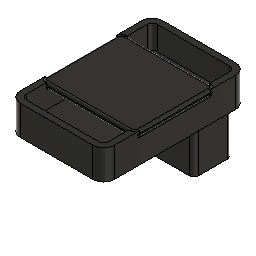
HX711mount (Autodesk Fusion 360 design; units mm, degrees)
Autodesk Fusion 360 part; units mm, degrees
sketch "Sketch1" plane through (0, 0, -6.0198) normal (0, 0, 1) x (-1, 0, 0)
  line L0 (-4.0409, -120.65) -> (2.9359, -120.65)
  line L1 (2.9359, -120.65) -> (3.9347, -119.6512)
  line L2 (3.9347, -119.6512) -> (3.9347, -58.1488)
  line L3 (3.9347, -58.1488) -> (2.9359, -57.15)
  line L4 (2.9359, -57.15) -> (3.9347, -56.1512)
  line L5 (3.9347, -56.1512) -> (3.9347, 6.35)
  line L6 (3.9347, 6.35) -> (-16.6393, 6.35)
  line L7 (-16.6393, 6.35) -> (-16.6393, -56.1512)
  line L8 (-16.6393, -56.1512) -> (-15.6405, -57.15)
  line L9 (-15.6405, -57.15) -> (-16.6393, -58.1488)
  line L10 (-16.6393, -58.1488) -> (-16.6393, -119.6512)
  line L11 (-16.6393, -119.6512) -> (-15.6405, -120.65)
  line L12 (-15.6405, -120.65) -> (-8.6637, -120.65)
  line L13 (-8.6637, -120.65) -> (-8.6637, -118.8466)
  arc A0 (-8.1557, -118.3386) -> (-8.6637, -118.8466) centre (-8.1557, -118.8466) ccw
  line L14 (-8.1557, -118.3386) -> (-4.5489, -118.3386)
  arc A1 (-4.0409, -118.8466) -> (-4.5489, -118.3386) centre (-4.5489, -118.8466) ccw
  line L15 (-4.0409, -118.8466) -> (-4.0409, -120.65)
  arc A2 (-8.1557, -105.6386) -> (-8.6637, -106.1466) centre (-8.1557, -106.1466) ccw
  line L16 (-8.1557, -105.6386) -> (-4.5489, -105.6386)
  arc A3 (-4.0409, -106.1466) -> (-4.5489, -105.6386) centre (-4.5489, -106.1466) ccw
  line L17 (-4.0409, -106.1466) -> (-4.0409, -109.7534)
  arc A4 (-4.5489, -110.2614) -> (-4.0409, -109.7534) centre (-4.5489, -109.7534) ccw
  line L18 (-4.5489, -110.2614) -> (-8.1557, -110.2614)
  arc A5 (-8.6637, -109.7534) -> (-8.1557, -110.2614) centre (-8.1557, -109.7534) ccw
  line L19 (-8.6637, -109.7534) -> (-8.6637, -106.1466)
  arc A6 (-8.1557, -92.9386) -> (-8.6637, -93.4466) centre (-8.1557, -93.4466) ccw
  line L20 (-8.1557, -92.9386) -> (-4.5489, -92.9386)
  arc A7 (-4.0409, -93.4466) -> (-4.5489, -92.9386) centre (-4.5489, -93.4466) ccw
  line L21 (-4.0409, -93.4466) -> (-4.0409, -97.0534)
  arc A8 (-4.5489, -97.5614) -> (-4.0409, -97.0534) centre (-4.5489, -97.0534) ccw
  line L22 (-4.5489, -97.5614) -> (-8.1557, -97.5614)
  arc A9 (-8.6637, -97.0534) -> (-8.1557, -97.5614) centre (-8.1557, -97.0534) ccw
  line L23 (-8.6637, -97.0534) -> (-8.6637, -93.4466)
  arc A10 (-8.1557, -80.2386) -> (-8.6637, -80.7466) centre (-8.1557, -80.7466) ccw
  line L24 (-8.1557, -80.2386) -> (-4.5489, -80.2386)
  arc A11 (-4.0409, -80.7466) -> (-4.5489, -80.2386) centre (-4.5489, -80.7466) ccw
  line L25 (-4.0409, -80.7466) -> (-4.0409, -84.3534)
  arc A12 (-4.5489, -84.8614) -> (-4.0409, -84.3534) centre (-4.5489, -84.3534) ccw
  line L26 (-4.5489, -84.8614) -> (-8.1557, -84.8614)
  arc A13 (-8.6637, -84.3534) -> (-8.1557, -84.8614) centre (-8.1557, -84.3534) ccw
  line L27 (-8.6637, -84.3534) -> (-8.6637, -80.7466)
  arc A14 (-8.1557, -67.5386) -> (-8.6637, -68.0466) centre (-8.1557, -68.0466) ccw
  line L28 (-8.1557, -67.5386) -> (-4.5489, -67.5386)
  arc A15 (-4.0409, -68.0466) -> (-4.5489, -67.5386) centre (-4.5489, -68.0466) ccw
  line L29 (-4.0409, -68.0466) -> (-4.0409, -71.6534)
  arc A16 (-4.5489, -72.1614) -> (-4.0409, -71.6534) centre (-4.5489, -71.6534) ccw
  line L30 (-4.5489, -72.1614) -> (-8.1557, -72.1614)
  arc A17 (-8.6637, -71.6534) -> (-8.1557, -72.1614) centre (-8.1557, -71.6534) ccw
  line L31 (-8.6637, -71.6534) -> (-8.6637, -68.0466)
  arc A18 (-8.1557, -54.8386) -> (-8.6637, -55.3466) centre (-8.1557, -55.3466) ccw
  line L32 (-8.1557, -54.8386) -> (-4.5489, -54.8386)
  arc A19 (-4.0409, -55.3466) -> (-4.5489, -54.8386) centre (-4.5489, -55.3466) ccw
  line L33 (-4.0409, -55.3466) -> (-4.0409, -58.9534)
  arc A20 (-4.5489, -59.4614) -> (-4.0409, -58.9534) centre (-4.5489, -58.9534) ccw
  line L34 (-4.5489, -59.4614) -> (-8.1557, -59.4614)
  arc A21 (-8.6637, -58.9534) -> (-8.1557, -59.4614) centre (-8.1557, -58.9534) ccw
  line L35 (-8.6637, -58.9534) -> (-8.6637, -55.3466)
  arc A22 (-8.1557, -42.1386) -> (-8.6637, -42.6466) centre (-8.1557, -42.6466) ccw
  line L36 (-8.1557, -42.1386) -> (-4.5489, -42.1386)
  arc A23 (-4.0409, -42.6466) -> (-4.5489, -42.1386) centre (-4.5489, -42.6466) ccw
  line L37 (-4.0409, -42.6466) -> (-4.0409, -46.2534)
  arc A24 (-4.5489, -46.7614) -> (-4.0409, -46.2534) centre (-4.5489, -46.2534) ccw
  line L38 (-4.5489, -46.7614) -> (-8.1557, -46.7614)
  arc A25 (-8.6637, -46.2534) -> (-8.1557, -46.7614) centre (-8.1557, -46.2534) ccw
  line L39 (-8.6637, -46.2534) -> (-8.6637, -42.6466)
  arc A26 (-8.1557, -29.4386) -> (-8.6637, -29.9466) centre (-8.1557, -29.9466) ccw
  line L40 (-8.1557, -29.4386) -> (-4.5489, -29.4386)
  arc A27 (-4.0409, -29.9466) -> (-4.5489, -29.4386) centre (-4.5489, -29.9466) ccw
  line L41 (-4.0409, -29.9466) -> (-4.0409, -33.5534)
  arc A28 (-4.5489, -34.0614) -> (-4.0409, -33.5534) centre (-4.5489, -33.5534) ccw
  line L42 (-4.5489, -34.0614) -> (-8.1557, -34.0614)
  arc A29 (-8.6637, -33.5534) -> (-8.1557, -34.0614) centre (-8.1557, -33.5534) ccw
  line L43 (-8.6637, -33.5534) -> (-8.6637, -29.9466)
  arc A30 (1.8011, -116.6114) -> (2.3091, -116.1034) centre (1.8011, -116.1034) ccw
  line L44 (1.8011, -116.6114) -> (-1.8057, -116.6114)
  arc A31 (-2.3137, -116.1034) -> (-1.8057, -116.6114) centre (-1.8057, -116.1034) ccw
  line L45 (-2.3137, -116.1034) -> (-2.3137, -112.4966)
  arc A32 (-1.8057, -111.9886) -> (-2.3137, -112.4966) centre (-1.8057, -112.4966) ccw
  line L46 (-1.8057, -111.9886) -> (1.8011, -111.9886)
  arc A33 (2.3091, -112.4966) -> (1.8011, -111.9886) centre (1.8011, -112.4966) ccw
  line L47 (2.3091, -112.4966) -> (2.3091, -116.1034)
  arc A34 (1.8011, -103.9114) -> (2.3091, -103.4034) centre (1.8011, -103.4034) ccw
  line L48 (1.8011, -103.9114) -> (-1.8057, -103.9114)
  arc A35 (-2.3137, -103.4034) -> (-1.8057, -103.9114) centre (-1.8057, -103.4034) ccw
  line L49 (-2.3137, -103.4034) -> (-2.3137, -99.7966)
  arc A36 (-1.8057, -99.2886) -> (-2.3137, -99.7966) centre (-1.8057, -99.7966) ccw
  line L50 (-1.8057, -99.2886) -> (1.8011, -99.2886)
  arc A37 (2.3091, -99.7966) -> (1.8011, -99.2886) centre (1.8011, -99.7966) ccw
  line L51 (2.3091, -99.7966) -> (2.3091, -103.4034)
  arc A38 (1.8011, -91.2114) -> (2.3091, -90.7034) centre (1.8011, -90.7034) ccw
  line L52 (1.8011, -91.2114) -> (-1.8057, -91.2114)
  arc A39 (-2.3137, -90.7034) -> (-1.8057, -91.2114) centre (-1.8057, -90.7034) ccw
  line L53 (-2.3137, -90.7034) -> (-2.3137, -87.0966)
  arc A40 (-1.8057, -86.5886) -> (-2.3137, -87.0966) centre (-1.8057, -87.0966) ccw
  line L54 (-1.8057, -86.5886) -> (1.8011, -86.5886)
  arc A41 (2.3091, -87.0966) -> (1.8011, -86.5886) centre (1.8011, -87.0966) ccw
  line L55 (2.3091, -87.0966) -> (2.3091, -90.7034)
  arc A42 (1.8011, -78.5114) -> (2.3091, -78.0034) centre (1.8011, -78.0034) ccw
  line L56 (1.8011, -78.5114) -> (-1.8057, -78.5114)
  arc A43 (-2.3137, -78.0034) -> (-1.8057, -78.5114) centre (-1.8057, -78.0034) ccw
  line L57 (-2.3137, -78.0034) -> (-2.3137, -74.3966)
  arc A44 (-1.8057, -73.8886) -> (-2.3137, -74.3966) centre (-1.8057, -74.3966) ccw
  line L58 (-1.8057, -73.8886) -> (1.8011, -73.8886)
  arc A45 (2.3091, -74.3966) -> (1.8011, -73.8886) centre (1.8011, -74.3966) ccw
  line L59 (2.3091, -74.3966) -> (2.3091, -78.0034)
  arc A46 (1.8011, -65.8114) -> (2.3091, -65.3034) centre (1.8011, -65.3034) ccw
  line L60 (1.8011, -65.8114) -> (-1.8057, -65.8114)
  arc A47 (-2.3137, -65.3034) -> (-1.8057, -65.8114) centre (-1.8057, -65.3034) ccw
  line L61 (-2.3137, -65.3034) -> (-2.3137, -61.6966)
  arc A48 (-1.8057, -61.1886) -> (-2.3137, -61.6966) centre (-1.8057, -61.6966) ccw
  line L62 (-1.8057, -61.1886) -> (1.8011, -61.1886)
  arc A49 (2.3091, -61.6966) -> (1.8011, -61.1886) centre (1.8011, -61.6966) ccw
  line L63 (2.3091, -61.6966) -> (2.3091, -65.3034)
  arc A50 (1.8011, -53.1114) -> (2.3091, -52.6034) centre (1.8011, -52.6034) ccw
  line L64 (1.8011, -53.1114) -> (-1.8057, -53.1114)
  arc A51 (-2.3137, -52.6034) -> (-1.8057, -53.1114) centre (-1.8057, -52.6034) ccw
  line L65 (-2.3137, -52.6034) -> (-2.3137, -48.9966)
  arc A52 (-1.8057, -48.4886) -> (-2.3137, -48.9966) centre (-1.8057, -48.9966) ccw
  line L66 (-1.8057, -48.4886) -> (1.8011, -48.4886)
  arc A53 (2.3091, -48.9966) -> (1.8011, -48.4886) centre (1.8011, -48.9966) ccw
  line L67 (2.3091, -48.9966) -> (2.3091, -52.6034)
  arc A54 (1.8011, -40.4114) -> (2.3091, -39.9034) centre (1.8011, -39.9034) ccw
  line L68 (1.8011, -40.4114) -> (-1.8057, -40.4114)
  arc A55 (-2.3137, -39.9034) -> (-1.8057, -40.4114) centre (-1.8057, -39.9034) ccw
  line L69 (-2.3137, -39.9034) -> (-2.3137, -36.2966)
  arc A56 (-1.8057, -35.7886) -> (-2.3137, -36.2966) centre (-1.8057, -36.2966) ccw
  line L70 (-1.8057, -35.7886) -> (1.8011, -35.7886)
  arc A57 (2.3091, -36.2966) -> (1.8011, -35.7886) centre (1.8011, -36.2966) ccw
  line L71 (2.3091, -36.2966) -> (2.3091, -39.9034)
  arc A58 (1.8011, -27.7114) -> (2.3091, -27.2034) centre (1.8011, -27.2034) ccw
  line L72 (1.8011, -27.7114) -> (-1.8057, -27.7114)
  arc A59 (-2.3137, -27.2034) -> (-1.8057, -27.7114) centre (-1.8057, -27.2034) ccw
  line L73 (-2.3137, -27.2034) -> (-2.3137, -23.5966)
  arc A60 (-1.8057, -23.0886) -> (-2.3137, -23.5966) centre (-1.8057, -23.5966) ccw
  line L74 (-1.8057, -23.0886) -> (1.8011, -23.0886)
  arc A61 (2.3091, -23.5966) -> (1.8011, -23.0886) centre (1.8011, -23.5966) ccw
  line L75 (2.3091, -23.5966) -> (2.3091, -27.2034)
  arc A62 (1.8011, -15.0114) -> (2.3091, -14.5034) centre (1.8011, -14.5034) ccw
  line L76 (1.8011, -15.0114) -> (-1.8057, -15.0114)
  arc A63 (-2.3137, -14.5034) -> (-1.8057, -15.0114) centre (-1.8057, -14.5034) ccw
  line L77 (-2.3137, -14.5034) -> (-2.3137, -10.8966)
  arc A64 (-1.8057, -10.3886) -> (-2.3137, -10.8966) centre (-1.8057, -10.8966) ccw
  line L78 (-1.8057, -10.3886) -> (1.8011, -10.3886)
  arc A65 (2.3091, -10.8966) -> (1.8011, -10.3886) centre (1.8011, -10.8966) ccw
  line L79 (2.3091, -10.8966) -> (2.3091, -14.5034)
  arc A66 (1.8011, -2.3114) -> (2.3091, -1.8034) centre (1.8011, -1.8034) ccw
  line L80 (1.8011, -2.3114) -> (-1.8057, -2.3114)
  arc A67 (-2.3137, -1.8034) -> (-1.8057, -2.3114) centre (-1.8057, -1.8034) ccw
  line L81 (-2.3137, -1.8034) -> (-2.3137, 1.8034)
  arc A68 (-1.8057, 2.3114) -> (-2.3137, 1.8034) centre (-1.8057, 1.8034) ccw
  line L82 (-1.8057, 2.3114) -> (1.8011, 2.3114)
  arc A69 (2.3091, 1.8034) -> (1.8011, 2.3114) centre (1.8011, 1.8034) ccw
  line L83 (2.3091, 1.8034) -> (2.3091, -1.8034)
  arc A70 (-10.8989, -116.6114) -> (-10.3909, -116.1034) centre (-10.8989, -116.1034) ccw
  line L84 (-10.8989, -116.6114) -> (-14.5057, -116.6114)
  arc A71 (-15.0137, -116.1034) -> (-14.5057, -116.6114) centre (-14.5057, -116.1034) ccw
  line L85 (-15.0137, -116.1034) -> (-15.0137, -112.4966)
  arc A72 (-14.5057, -111.9886) -> (-15.0137, -112.4966) centre (-14.5057, -112.4966) ccw
  line L86 (-14.5057, -111.9886) -> (-10.8989, -111.9886)
  arc A73 (-10.3909, -112.4966) -> (-10.8989, -111.9886) centre (-10.8989, -112.4966) ccw
  line L87 (-10.3909, -112.4966) -> (-10.3909, -116.1034)
  arc A74 (-10.8989, -103.9114) -> (-10.3909, -103.4034) centre (-10.8989, -103.4034) ccw
  line L88 (-10.8989, -103.9114) -> (-14.5057, -103.9114)
  arc A75 (-15.0137, -103.4034) -> (-14.5057, -103.9114) centre (-14.5057, -103.4034) ccw
  line L89 (-15.0137, -103.4034) -> (-15.0137, -99.7966)
  arc A76 (-14.5057, -99.2886) -> (-15.0137, -99.7966) centre (-14.5057, -99.7966) ccw
  line L90 (-14.5057, -99.2886) -> (-10.8989, -99.2886)
  arc A77 (-10.3909, -99.7966) -> (-10.8989, -99.2886) centre (-10.8989, -99.7966) ccw
  line L91 (-10.3909, -99.7966) -> (-10.3909, -103.4034)
  arc A78 (-10.8989, -91.2114) -> (-10.3909, -90.7034) centre (-10.8989, -90.7034) ccw
  line L92 (-10.8989, -91.2114) -> (-14.5057, -91.2114)
  arc A79 (-15.0137, -90.7034) -> (-14.5057, -91.2114) centre (-14.5057, -90.7034) ccw
  line L93 (-15.0137, -90.7034) -> (-15.0137, -87.0966)
  arc A80 (-14.5057, -86.5886) -> (-15.0137, -87.0966) centre (-14.5057, -87.0966) ccw
  line L94 (-14.5057, -86.5886) -> (-10.8989, -86.5886)
  arc A81 (-10.3909, -87.0966) -> (-10.8989, -86.5886) centre (-10.8989, -87.0966) ccw
  line L95 (-10.3909, -87.0966) -> (-10.3909, -90.7034)
  arc A82 (-10.8989, -78.5114) -> (-10.3909, -78.0034) centre (-10.8989, -78.0034) ccw
  line L96 (-10.8989, -78.5114) -> (-14.5057, -78.5114)
  arc A83 (-15.0137, -78.0034) -> (-14.5057, -78.5114) centre (-14.5057, -78.0034) ccw
  line L97 (-15.0137, -78.0034) -> (-15.0137, -74.3966)
  arc A84 (-14.5057, -73.8886) -> (-15.0137, -74.3966) centre (-14.5057, -74.3966) ccw
  line L98 (-14.5057, -73.8886) -> (-10.8989, -73.8886)
  arc A85 (-10.3909, -74.3966) -> (-10.8989, -73.8886) centre (-10.8989, -74.3966) ccw
  line L99 (-10.3909, -74.3966) -> (-10.3909, -78.0034)
  arc A86 (-10.8989, -65.8114) -> (-10.3909, -65.3034) centre (-10.8989, -65.3034) ccw
  line L100 (-10.8989, -65.8114) -> (-14.5057, -65.8114)
  arc A87 (-15.0137, -65.3034) -> (-14.5057, -65.8114) centre (-14.5057, -65.3034) ccw
  line L101 (-15.0137, -65.3034) -> (-15.0137, -61.6966)
  arc A88 (-14.5057, -61.1886) -> (-15.0137, -61.6966) centre (-14.5057, -61.6966) ccw
  line L102 (-14.5057, -61.1886) -> (-10.8989, -61.1886)
  arc A89 (-10.3909, -61.6966) -> (-10.8989, -61.1886) centre (-10.8989, -61.6966) ccw
  line L103 (-10.3909, -61.6966) -> (-10.3909, -65.3034)
  arc A90 (-10.8989, -53.1114) -> (-10.3909, -52.6034) centre (-10.8989, -52.6034) ccw
  line L104 (-10.8989, -53.1114) -> (-14.5057, -53.1114)
  arc A91 (-15.0137, -52.6034) -> (-14.5057, -53.1114) centre (-14.5057, -52.6034) ccw
  line L105 (-15.0137, -52.6034) -> (-15.0137, -48.9966)
  arc A92 (-14.5057, -48.4886) -> (-15.0137, -48.9966) centre (-14.5057, -48.9966) ccw
  line L106 (-14.5057, -48.4886) -> (-10.8989, -48.4886)
  arc A93 (-10.3909, -48.9966) -> (-10.8989, -48.4886) centre (-10.8989, -48.9966) ccw
  line L107 (-10.3909, -48.9966) -> (-10.3909, -52.6034)
  arc A94 (-10.8989, -40.4114) -> (-10.3909, -39.9034) centre (-10.8989, -39.9034) ccw
  line L108 (-10.8989, -40.4114) -> (-14.5057, -40.4114)
  arc A95 (-15.0137, -39.9034) -> (-14.5057, -40.4114) centre (-14.5057, -39.9034) ccw
  line L109 (-15.0137, -39.9034) -> (-15.0137, -36.2966)
  arc A96 (-14.5057, -35.7886) -> (-15.0137, -36.2966) centre (-14.5057, -36.2966) ccw
  line L110 (-14.5057, -35.7886) -> (-10.8989, -35.7886)
  arc A97 (-10.3909, -36.2966) -> (-10.8989, -35.7886) centre (-10.8989, -36.2966) ccw
  line L111 (-10.3909, -36.2966) -> (-10.3909, -39.9034)
  arc A98 (-10.8989, -27.7114) -> (-10.3909, -27.2034) centre (-10.8989, -27.2034) ccw
  line L112 (-10.8989, -27.7114) -> (-14.5057, -27.7114)
  arc A99 (-15.0137, -27.2034) -> (-14.5057, -27.7114) centre (-14.5057, -27.2034) ccw
  line L113 (-15.0137, -27.2034) -> (-15.0137, -23.5966)
  arc A100 (-14.5057, -23.0886) -> (-15.0137, -23.5966) centre (-14.5057, -23.5966) ccw
  line L114 (-14.5057, -23.0886) -> (-10.8989, -23.0886)
  arc A101 (-10.3909, -23.5966) -> (-10.8989, -23.0886) centre (-10.8989, -23.5966) ccw
  line L115 (-10.3909, -23.5966) -> (-10.3909, -27.2034)
  arc A102 (-10.8989, -15.0114) -> (-10.3909, -14.5034) centre (-10.8989, -14.5034) ccw
  line L116 (-10.8989, -15.0114) -> (-14.5057, -15.0114)
  arc A103 (-15.0137, -14.5034) -> (-14.5057, -15.0114) centre (-14.5057, -14.5034) ccw
  line L117 (-15.0137, -14.5034) -> (-15.0137, -10.8966)
  arc A104 (-14.5057, -10.3886) -> (-15.0137, -10.8966) centre (-14.5057, -10.8966) ccw
  line L118 (-14.5057, -10.3886) -> (-10.8989, -10.3886)
  arc A105 (-10.3909, -10.8966) -> (-10.8989, -10.3886) centre (-10.8989, -10.8966) ccw
  line L119 (-10.3909, -10.8966) -> (-10.3909, -14.5034)
  arc A106 (-10.8989, -2.3114) -> (-10.3909, -1.8034) centre (-10.8989, -1.8034) ccw
  line L120 (-10.8989, -2.3114) -> (-14.5057, -2.3114)
  arc A107 (-15.0137, -1.8034) -> (-14.5057, -2.3114) centre (-14.5057, -1.8034) ccw
  line L121 (-15.0137, -1.8034) -> (-15.0137, 1.8034)
  arc A108 (-14.5057, 2.3114) -> (-15.0137, 1.8034) centre (-14.5057, 1.8034) ccw
  line L122 (-14.5057, 2.3114) -> (-10.8989, 2.3114)
  arc A109 (-10.3909, 1.8034) -> (-10.8989, 2.3114) centre (-10.8989, 1.8034) ccw
  line L123 (-10.3909, 1.8034) -> (-10.3909, -1.8034)
  arc A110 (-8.6637, -8.1534) -> (-8.1557, -8.6614) centre (-8.1557, -8.1534) ccw
  line L124 (-8.6637, -8.1534) -> (-8.6637, -4.5466)
  arc A111 (-8.1557, -4.0386) -> (-8.6637, -4.5466) centre (-8.1557, -4.5466) ccw
  line L125 (-8.1557, -4.0386) -> (-4.5489, -4.0386)
  arc A112 (-4.0409, -4.5466) -> (-4.5489, -4.0386) centre (-4.5489, -4.5466) ccw
  line L126 (-4.0409, -4.5466) -> (-4.0409, -8.1534)
  arc A113 (-4.5489, -8.6614) -> (-4.0409, -8.1534) centre (-4.5489, -8.1534) ccw
  line L127 (-4.5489, -8.6614) -> (-8.1557, -8.6614)
  arc A114 (-8.1557, -16.7386) -> (-8.6637, -17.2466) centre (-8.1557, -17.2466) ccw
  line L128 (-8.1557, -16.7386) -> (-4.5489, -16.7386)
  arc A115 (-4.0409, -17.2466) -> (-4.5489, -16.7386) centre (-4.5489, -17.2466) ccw
  line L129 (-4.0409, -17.2466) -> (-4.0409, -20.8534)
  arc A116 (-4.5489, -21.3614) -> (-4.0409, -20.8534) centre (-4.5489, -20.8534) ccw
  line L130 (-4.5489, -21.3614) -> (-8.1557, -21.3614)
  arc A117 (-8.6637, -20.8534) -> (-8.1557, -21.3614) centre (-8.1557, -20.8534) ccw
  line L131 (-8.6637, -20.8534) -> (-8.6637, -17.2466)
  line L132 (2.6647, -119.6512) -> (-15.3693, -119.6512)
  line L133 (-16.6393, -118.3812) -> (-16.6393, -110.7612)
  line L134 (-15.3693, -109.4912) -> (2.6647, -109.4912)
  line L135 (3.9347, -110.7612) -> (3.9347, -118.3812)
  arc A118 (-16.6393, -118.3812) -> (-15.3693, -119.6512) centre (-15.3693, -118.3812) ccw
  arc A119 (-15.3693, -109.4912) -> (-16.6393, -110.7612) centre (-15.3693, -110.7612) ccw
  arc A120 (3.9347, -110.7612) -> (2.6647, -109.4912) centre (2.6647, -110.7612) ccw
  arc A121 (2.6647, -119.6512) -> (3.9347, -118.3812) centre (2.6647, -118.3812) ccw
  point P0 (-16.6393, -119.6512)
  point P1 (-16.6393, -109.4912)
  dimension "d1" = 10.16
  dimension "d2" = 1.27
  constraint coincident P0 L10.end
  constraint coincident L10 P1
  constraint perpendicular L2 L134
  constraint coincident P0 L132
  constraint coincident P0 L133
  constraint tangent L132 A118
  constraint tangent L133 A118
  constraint coincident P1 L133
  constraint coincident P1 L134
  constraint tangent L133 A119
  constraint tangent L134 A119
  constraint equal A118 A119
  constraint tangent L134 A120
  constraint tangent L135 A120
  constraint equal A118 A120
  constraint tangent L132 A121
  constraint tangent L135 A121
  constraint equal A118 A121
  measures "d1" distance of P0 P1
  measures "d2" radius of A118
extrude "Extrude1" add sketch "Sketch1" along normal blind 12.7 contours L13 A0 L14 A1 L15 L132 | L2 L10 L13 A0 L14 A1 L15 L17 A4 L18 A5 L19 L132 L133 L134 L135 A118 A119 A120 A121 | L17 A4 L18 A5 L19 L134 | A30 L44 A31 L45 A32 L46 A33 L47 | A70 L84 A71 L85 A72 L86 A73 L87 makes body 1
sketch "Sketch2" plane through (0, 0, 6.6802) normal (0, 0, 1) x (-1, 0, 0)
  arc A0 (-16.6393, -118.3812) -> (-15.3693, -119.6512) centre (-15.3693, -118.3812) ccw
  line L0 (-15.3693, -119.6512) -> (2.6647, -119.6512)
  arc A1 (2.6647, -119.6512) -> (3.9347, -118.3812) centre (2.6647, -118.3812) ccw
  line L1 (3.9347, -118.3812) -> (3.9347, -110.7612)
  arc A2 (3.9347, -110.7612) -> (2.6647, -109.4912) centre (2.6647, -110.7612) ccw
  line L2 (2.6647, -109.4912) -> (-15.3693, -109.4912)
  arc A3 (-15.3693, -109.4912) -> (-16.6393, -110.7612) centre (-15.3693, -110.7612) ccw
  line L3 (-16.6393, -110.7612) -> (-16.6393, -118.3812)
  line L4 (-6.3523, -119.6512) -> (3.3777, -119.6512)
  line L5 (-6.3523, -119.6512) -> (-16.0823, -119.6512)
  line L6 (-17.3523, -118.3812) -> (-17.3523, -85.9212)
  line L7 (-16.0823, -84.6512) -> (3.3777, -84.6512)
  line L8 (4.6477, -85.9212) -> (4.6477, -118.3812)
  arc A4 (3.3777, -119.6512) -> (4.6477, -118.3812) centre (3.3777, -118.3812) ccw
  arc A5 (-17.3523, -118.3812) -> (-16.0823, -119.6512) centre (-16.0823, -118.3812) ccw
  arc A6 (-16.0823, -84.6512) -> (-17.3523, -85.9212) centre (-16.0823, -85.9212) ccw
  arc A7 (4.6477, -85.9212) -> (3.3777, -84.6512) centre (3.3777, -85.9212) ccw
  arc A8 (3.3777, -121.2387) -> (6.2352, -118.3812) centre (3.3777, -118.3812) ccw
  line L9 (6.2352, -85.9212) -> (6.2352, -118.3812)
  arc A9 (6.2352, -85.9212) -> (3.3777, -83.0637) centre (3.3777, -85.9212) ccw
  line L10 (-16.0823, -83.0637) -> (3.3777, -83.0637)
  arc A10 (-16.0823, -83.0637) -> (-18.9398, -85.9212) centre (-16.0823, -85.9212) ccw
  line L11 (-18.9398, -118.3812) -> (-18.9398, -85.9212)
  arc A11 (-18.9398, -118.3812) -> (-16.0823, -121.2387) centre (-16.0823, -118.3812) ccw
  line L12 (-6.3523, -121.2387) -> (-16.0823, -121.2387)
  line L13 (-6.3523, -121.2387) -> (3.3777, -121.2387)
  point P0 (4.6477, -119.6512)
  point P1 (-17.3523, -119.6512)
  point P2 (-17.3523, -84.6512)
  point P3 (4.6477, -84.6512)
  dimension "d5" = 11
  dimension "d6" = 11
  dimension "d7" = 35
  dimension "d8" = 22
  dimension "d9" = 1.27
  dimension "d10" = -1.5875
  constraint midpoint L0 L4.start
  constraint parallel L0 L4
  constraint parallel L0 L5
  constraint perpendicular L5 L6
  constraint perpendicular L1 L7
  constraint coincident P0 L4
  constraint coincident P0 L8
  constraint tangent L4 A4
  constraint tangent L8 A4
  constraint coincident P1 L5
  constraint coincident P1 L6
  constraint tangent L5 A5
  constraint tangent L6 A5
  constraint equal A4 A5
  constraint coincident P2 L6
  constraint coincident P2 L7
  constraint tangent L6 A6
  constraint tangent L7 A6
  constraint equal A4 A6
  constraint coincident P3 L7
  constraint coincident P3 L8
  constraint tangent L7 A7
  constraint tangent L8 A7
  constraint equal A4 A7
  measures "d5" distance of L4.start P0
  measures "d6" distance of L4.start P1
  measures "d7" distance of P1 P2
  measures "d8" distance of P2 P3
  measures "d9" radius of A4
extrude "Extrude10" add sketch "Sketch2" along normal blind 6.35 separate body makes body 2
extrude "Extrude11" add sketch "Sketch2" along normal blind 1.5875 contours A0 L0 A1 L1 A2 L2 A3 L3 L4 L5 | A0 A1 L1 A2 L2 A3 L3 L4 L5 L6 L7 L8 A4 A5 A6 A7 bodies 1 2
extrude "Extrude12" add 1 faces at (6.3523, 120.1804, 13.0302) along direction (0, 0, 1) blind 1.5875 on bodies 1 bodies 1
sketch "Sketch10" plane through (0, 0, 14.6177) normal (0, 0, 1) x (-1, 0, 0)
  line L0 (3.3777, -119.6512) -> (-16.0823, -119.6512)
  arc A0 (-17.3523, -118.3812) -> (-16.0823, -119.6512) centre (-16.0823, -118.3812) ccw
  line L1 (-17.3523, -118.3812) -> (-17.3523, -85.9212)
  arc A1 (-16.0823, -84.6512) -> (-17.3523, -85.9212) centre (-16.0823, -85.9212) ccw
  line L2 (-16.0823, -84.6512) -> (3.3777, -84.6512)
  arc A2 (4.6477, -85.9212) -> (3.3777, -84.6512) centre (3.3777, -85.9212) ccw
  line L3 (4.6477, -85.9212) -> (4.6477, -118.3812)
  arc A3 (3.3777, -119.6512) -> (4.6477, -118.3812) centre (3.3777, -118.3812) ccw
  arc A4 (-18.9398, -118.3812) -> (-16.0823, -121.2387) centre (-16.0823, -118.3812) ccw
  line L4 (-16.0823, -121.2387) -> (3.3777, -121.2387)
  arc A5 (3.3777, -121.2387) -> (6.2352, -118.3812) centre (3.3777, -118.3812) ccw
  line L5 (6.2352, -118.3812) -> (6.2352, -85.9212)
  arc A6 (6.2352, -85.9212) -> (3.3777, -83.0637) centre (3.3777, -85.9212) ccw
  line L6 (3.3777, -83.0637) -> (-16.0823, -83.0637)
  arc A7 (-16.0823, -83.0637) -> (-18.9398, -85.9212) centre (-16.0823, -85.9212) ccw
  line L7 (-18.9398, -85.9212) -> (-18.9398, -118.3812)
  line L8 (-18.9398, -102.1512) -> (6.2352, -102.1512)
  line L9 (6.2352, -102.1512) -> (6.2352, -111.6762)
  line L10 (4.9652, -112.9462) -> (-17.6698, -112.9462)
  line L11 (-18.9398, -111.6762) -> (-18.9398, -92.6262)
  line L12 (-17.6698, -91.3562) -> (4.9652, -91.3562)
  line L13 (6.2352, -92.6262) -> (6.2352, -102.1512)
  arc A8 (4.9652, -112.9462) -> (6.2352, -111.6762) centre (4.9652, -111.6762) ccw
  arc A9 (-18.9398, -111.6762) -> (-17.6698, -112.9462) centre (-17.6698, -111.6762) ccw
  arc A10 (-17.6698, -91.3562) -> (-18.9398, -92.6262) centre (-17.6698, -92.6262) ccw
  arc A11 (6.2352, -92.6262) -> (4.9652, -91.3562) centre (4.9652, -92.6262) ccw
  point P0 (6.2352, -112.9462)
  point P1 (-18.9398, -112.9462)
  point P2 (-18.9398, -91.3562)
  dimension "d54" = 10.795
  dimension "d55" = 21.59
  dimension "d56" = 1.27
  constraint horizontal L8
  constraint midpoint L7 L8.start
  constraint coincident L5 L8.end
  constraint coincident L5 P0
  constraint coincident L7 P1
  constraint perpendicular L7 L10
  constraint coincident L7 P2
  constraint perpendicular L5 L12
  constraint coincident P0 L9
  constraint coincident P0 L10
  constraint tangent L9 A8
  constraint tangent L10 A8
  constraint coincident P1 L10
  constraint coincident P1 L11
  constraint tangent L10 A9
  constraint tangent L11 A9
  constraint equal A8 A9
  constraint coincident P2 L11
  constraint coincident P2 L12
  constraint tangent L11 A10
  constraint tangent L12 A10
  constraint equal A8 A10
  constraint tangent L12 A11
  constraint tangent L13 A11
  constraint equal A8 A11
  measures "d54" distance of L8.end P0
  measures "d55" distance of P1 P2
  measures "d56" radius of A8
extrude "Extrude13" cut sketch "Sketch10" against normal blind 1.5875 contours L3 L5 L8 L9 L10 A8 | L1 L7 L8 L10 L11 A9 | L3 L5 L8 L12 L13 A11 | L1 L7 L8 L11 L12 A10 bodies 1
extrude "Extrude14" add sketch "Sketch10" along normal blind 1.5875 separate body contours L1 L3 L8 L10 | L3 L5 L8 L9 L10 A8 | L1 L7 L8 L10 L11 A9 | L1 L3 L8 L12 | L3 L5 L8 L12 L13 A11 | L1 L7 L8 L11 L12 A10 makes body 3
fillet "Fillet2" radius 0.635 16 edges at (18.9398, 102.1512, 16.2052) (18.5678, 112.5742, 16.2052) (6.3523, 112.9462, 16.2052) (-5.8632, 112.5742, 16.2052) (-6.2352, 102.1512, 16.2052) (-5.8632, 91.7282, 16.2052) (6.3523, 91.3562, 16.2052) (18.5678, 91.7282, 16.2052) (-5.8632, 91.7282, 14.6177) (-6.2352, 102.1512, 14.6177) (-5.8632, 112.5742, 14.6177) (6.3523, 112.9462, 14.6177) (18.5678, 112.5742, 14.6177) (18.9398, 102.1512, 14.6177) (18.5678, 91.7282, 14.6177) (6.3523, 91.3562, 14.6177) on bodies 3
hole "Hole3" at (12.7, 114.3, -6.0198) direction (0, 0, 1) diameter 3.429 depth 9.525 tip angle 180 bodies 1
thread "Thread3" "ANSI Unified Screw Threads 0.164(#8) 8-32 UNC 8-32 UNC 2B" major diameter 4.1656 minor diameter 3.4163 pitch 0.7937 angle 60 modelled right hand crest width 0.2341 on face at (10.986, 114.2573, -2.8448) crest through (10.9919, 114.3, -5.8214) on bodies 1
hole "Hole4" at (0, 114.3, -6.0198) direction (0, 0, 1) diameter 3.429 depth 9.525 tip angle 180 bodies 1
thread "Thread4" "ANSI Unified Screw Threads 0.164(#8) 8-32 UNC 8-32 UNC 2B" major diameter 4.1656 minor diameter 3.4163 pitch 0.7937 angle 60 modelled right hand crest width 0.2341 on face at (-1.714, 114.2573, -2.8448) crest through (-1.7081, 114.3, -5.8214) on bodies 1
move_body "Move3" bodies 3 to x (1, 0, 0) y (0, 1, 0) z (0, 0, 1) at (0, 0, -1.5875)
equation "d10 = ( -0.125 / 2 ) * 1 in"
equation "d48 = ( 1 / 4 ) * 1 in"
equation "d50 = ( 1 / 16 ) * 1 in"
equation "d52 = ( 1 / 16 ) * 1 in"
equation "d57 = ( -1 / 16 ) * 1 in"
equation "d59 = ( 1 / 16 ) * 1 in"
named bodies: "HX711mount", "HX711cover"
